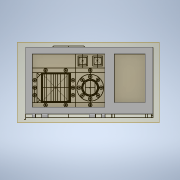
# Autodesk Inventor part: authentication panel v1.1
Saved by Autodesk Inventor 2022 (Build 260153000, 153)
## iProperties
Created: 2022-05-25
Part Number: authentication panel v1.1
Material: Generic
Document SubType Name: Modeling
Designer: alecw
Density: 1 g/cm^3
Appearance: Default
Author: alecw
Autodesk Inventor part; units mm, degrees
ref_plane "YZ Plane" through (0, 0, 0) normal (1, 0, 0) x (0, 1, 0)
ref_plane "XZ Plane" through (0, 0, 0) normal (0, 1, 0) x (-1, 0, 0)
ref_plane "Backplate Depth" through (0, 0, -3.2) normal (0, 0, 1) x (1, 0, 0)
sketch "Sketch2" plane through (0, 0, 0) normal (0, 0, 1) x (1, 0, 0)
  line L0 (0, 0) -> (45, 0)
  line L1 (45, 0) -> (45, 65)
  line L2 (45, 65) -> (0, 65)
  line L3 (0, 65) -> (0, 0)
  line L4 (0, 0) -> (-8.8, 0)
  line L5 (-8.8, 0) -> (-12, 0)
  line L6 (-12, 0) -> (-42, 0)
  line L7 (-42, 0) -> (-54.8, 0)
  line L8 (-54.8, 0) -> (-99.5, 0)
  line L9 (-99.5, 0) -> (-105.9, 0)
  line L10 (-105.9, 0) -> (-114.7, 0)
  line L11 (-114.7, 0) -> (-114.7, 40.1)
  line L12 (-114.7, 40.1) -> (0, 40.1)
  line L13 (-114.7, 0) -> (0, 0)
  line L14 (-105.9, 0) -> (-105.9, 40.1)
  line L15 (-8.8, 40.1) -> (-8.8, 0)
  line L16 (-48.4, 0) -> (-8.8, 0)
  line L17 (0, 65) -> (-114.7, 65)
  line L18 (-114.7, 65) -> (-114.7, 40.1)
  line L19 (45, 0) -> (48.2, 0)
  line L20 (0, 65) -> (0, 68.2)
  line L21 (0, 68.2) -> (48.2, 68.2)
  line L22 (48.2, 68.2) -> (48.2, 0)
  line L23 (-54.8, 0) -> (-48.4, 0)
  line L24 (-42, 0) -> (-48.4, 0)
  line L25 (-48.4, 0) -> (-48.4, 40.1)
  line L26 (-105.9, 40.1) -> (-105.9, 33.7)
  line L27 (-105.9, 40.1) -> (-93.1, 40.1)
  line L28 (-105.9, 0) -> (-48.4, 0)
  line L29 (-99.5, 0) -> (-88.19, 0)
  line L30 (-88.19, 0) -> (-79.22, 0)
  line L31 (-54.8, 0) -> (-54.8, 40.1)
  line L32 (-99.5, 0) -> (-99.5, 40.1)
  line L33 (-54.8, 40.1) -> (-56.9213, 37.9787)
  line L34 (-54.8, 40.1) -> (-51.8, 40.1) construction
  line L35 (-56.9213, 37.9787) -> (-54.8, 35.8574)
  line L36 (-56.9213, 37.9787) -> (-59.0426, 40.1)
  line L37 (-54.8, 0) -> (-57.6284, 2.8284)
  line L38 (-54.8, 0) -> (-50.8, 0) construction
  line L39 (-99.5, 40.1) -> (-95.9645, 36.5645)
  line L40 (-99.5, 40.1) -> (-94.5, 40.1) construction
  line L41 (-95.9645, 36.5645) -> (-92.4289, 40.1)
  line L42 (-95.9645, 36.5645) -> (-99.5, 33.0289)
  line L43 (-99.5, 0) -> (-95.9645, 3.5355)
  line L44 (-99.5, 0) -> (-94.5, 0) construction
  line L45 (-95.9645, 3.5355) -> (-92.4289, 0)
  line L46 (-95.9645, 3.5355) -> (-99.5, 7.0711)
  line L47 (-48.4, 0) -> (-48.4, -6.4)
  line L48 (-48.4, -6.4) -> (-105.9, -6.4)
  line L49 (-105.9, -6.4) -> (-105.9, 0)
  line L50 (-105.9, 40.1) -> (-105.9, 46.5)
  line L51 (-48.4, 40.1) -> (-48.4, 46.5)
  line L52 (-48.4, 46.5) -> (-105.9, 46.5)
  line L53 (-88.19, 0) -> (-86.59, 0)
  line L54 (-88.19, 0) -> (-89.79, 0)
  line L55 (-89.79, 0) -> (-86.59, 0)
  line L56 (-86.59, 0) -> (-86.59, 40.1)
  line L57 (-86.59, 40.1) -> (-89.79, 40.1)
  line L58 (-89.79, 40.1) -> (-89.79, 0)
  line L59 (-80.82, 40.1) -> (-80.82, 0)
  line L60 (-77.62, 0) -> (-77.62, 40.1)
  line L61 (-71.85, 40.1) -> (-71.85, 0)
  line L62 (-68.65, 0) -> (-68.65, 40.1)
  line L63 (-62.88, 40.1) -> (-62.88, 0)
  line L64 (-59.68, 0) -> (-59.68, 40.1)
  line L65 (0, 0) -> (0, -6.4)
  line L66 (0, -6.4) -> (0, -15.2)
  line L67 (-114.7, 0) -> (-114.7, -6.4)
  line L68 (-114.7, -6.4) -> (-114.7, -15.2)
  line L69 (-114.7, -15.2) -> (0, -15.2)
  line L70 (0, -15.2) -> (48.2, -15.2)
  line L71 (48.2, -15.2) -> (48.2, 0)
  line L72 (-28.6, 40.1) -> (-28.6, 0)
  circle A0 centre (-28.6, 20.05) radius 9.5
  circle A1 centre (-28.6, 20.05) radius 10.5
  line L73 (-28.6, 29.55) -> (-27.4024, 29.4742)
  line L74 (-27.4024, 29.4742) -> (-27.3391, 30.474)
  line L75 (-28.6, 29.55) -> (-29.7976, 29.4742)
  line L76 (-29.7976, 29.4742) -> (-29.8609, 30.474)
  line L77 (-105.9, 46.5) -> (-114.7, 46.5)
  line L78 (-105.9, -6.4) -> (-114.7, -6.4)
  line L79 (-48.4, -6.4) -> (0, -6.4)
  line L80 (-28.6, 20.05) -> (-35, 20.05)
  line L81 (-28.6, 20.05) -> (-22.2, 20.05)
  circle A2 centre (-28.6, 20.05) radius 17.9
  line L82 (-77.62, 40.1) -> (-71.85, 40.1)
  line L83 (-88.19, 40.1) -> (-92.19, 40.1)
  line L84 (-92.19, 40.1) -> (-93.79, 40.1)
  line L85 (-74.735, 0) -> (-74.735, 40.1)
  line L86 (-92.135, 38.25) -> (-57.335, 38.25)
  line L87 (-57.335, 38.25) -> (-57.335, 1.85)
  line L88 (-57.335, 1.85) -> (-92.135, 1.85)
  line L89 (-92.135, 1.85) -> (-92.135, 38.25)
  line L90 (-92.135, 38.25) -> (-57.335, 1.85) construction
  line L91 (-57.335, 38.25) -> (-92.135, 1.85) construction
  line L92 (-74.735, 38.25) -> (-74.735, 40.1)
  line L93 (-18.1, 20.05) -> (-17.1, 20.05)
  circle A3 centre (-28.6, 20.05) radius 11.5
  line L94 (-17.1, 20.05) -> (-10.7, 20.05)
  circle A4 centre (-13.9, 20.05) radius 0.9
  line L95 (-54.8, 40.1) -> (-48.4, 40.1)
  line L96 (-89.79, 38.25) -> (-86.59, 38.25)
  line L97 (-59.68, 38.25) -> (-62.88, 38.25)
  line L98 (-92.135, 20.05) -> (-57.335, 20.05)
  circle A5 centre (-18.2055, 30.4445) radius 0.9
  circle A6 centre (-28.6, 34.75) radius 0.9
  circle A7 centre (-38.9945, 30.4445) radius 0.9
  circle A8 centre (-43.3, 20.05) radius 0.9
  circle A9 centre (-38.9945, 9.6555) radius 0.9
  circle A10 centre (-28.6, 5.35) radius 0.9
  circle A11 centre (-18.2055, 9.6555) radius 0.9
  line L99 (-57.6284, 2.8284) -> (-54.8, 5.6569)
  line L100 (-57.6284, 2.8284) -> (-60.4569, 0)
  line L101 (-99.5, 20.05) -> (-105.9, 20.05)
  circle A12 centre (-102.7, 20.05) radius 0.9
  line L102 (-54.8, 20.05) -> (-48.4, 20.05)
  circle A13 centre (-51.6, 20.05) radius 0.9
  line L103 (0, -15.2) -> (0, -20)
  line L104 (0, -20) -> (-114.7, -20)
  line L105 (-114.7, -20) -> (-114.7, -15.2)
  line L106 (-88.19, 40.1) -> (-88.19, 43.3)
  circle A14 centre (-88.19, 43.3) radius 0.9
  circle A15 centre (-61.28, 43.3) radius 0.9
  circle A16 centre (-88.19, -3.2) radius 0.9
  circle A17 centre (-61.28, -3.2) radius 0.9
  line L107 (-102.7, 20.05) -> (-102.7, 0)
  circle A18 centre (-102.7, 10.025) radius 0.9
  circle A19 centre (-102.7, 30.075) radius 0.9
  circle A20 centre (-51.6, 30.075) radius 0.9
  circle A21 centre (-51.6, 10.025) radius 0.9
  line L108 (0, -20) -> (48.2, -20)
  line L109 (48.2, -20) -> (48.2, -15.2)
  line L110 (0, 65) -> (0, 73.8)
  line L111 (0, 73.8) -> (-114.7, 73.8)
  line L112 (-114.7, 73.8) -> (-114.7, 65)
  line L113 (-105.9, -20) -> (-105.9, 73.8)
  line L114 (-8.8, -20) -> (-8.8, 73.8)
  line L115 (-28.6, 40.1) -> (-48.4, 40.1)
  line L116 (-28.6, 40.1) -> (-8.8, 40.1)
  line L117 (-48.4, 46.5) -> (-28.6, 46.5)
  line L118 (-28.6, 46.5) -> (-8.8, 46.5)
  line L119 (-38.5, 46.5) -> (-38.5, 65)
  line L120 (-18.7, 46.5) -> (-18.7, 65)
  line L121 (-13.7, 60.75) -> (-23.7, 60.75)
  line L122 (-23.7, 60.75) -> (-23.7, 50.75)
  line L123 (-23.7, 50.75) -> (-13.7, 50.75)
  line L124 (-13.7, 50.75) -> (-13.7, 60.75)
  line L125 (-13.7, 60.75) -> (-23.7, 50.75) construction
  line L126 (-23.7, 60.75) -> (-13.7, 50.75) construction
  line L127 (-33.5, 50.75) -> (-43.5, 50.75)
  line L128 (-43.5, 50.75) -> (-43.5, 60.75)
  line L129 (-43.5, 60.75) -> (-33.5, 60.75)
  line L130 (-33.5, 60.75) -> (-33.5, 50.75)
  line L131 (-33.5, 50.75) -> (-43.5, 60.75) construction
  line L132 (-43.5, 50.75) -> (-33.5, 60.75) construction
  line L133 (-32, 49.25) -> (-45, 49.25)
  line L134 (-45, 49.25) -> (-45, 62.25)
  line L135 (-45, 62.25) -> (-32, 62.25)
  line L136 (-32, 62.25) -> (-32, 49.25)
  line L137 (-32, 49.25) -> (-45, 62.25) construction
  line L138 (-45, 49.25) -> (-32, 62.25) construction
  line L139 (-12.2, 62.25) -> (-25.2, 62.25)
  line L140 (-25.2, 62.25) -> (-25.2, 49.25)
  line L141 (-25.2, 49.25) -> (-12.2, 49.25)
  line L142 (-12.2, 49.25) -> (-12.2, 62.25)
  line L143 (-12.2, 62.25) -> (-25.2, 49.25) construction
  line L144 (-25.2, 62.25) -> (-12.2, 49.25) construction
  line L145 (-33.5, 50.75) -> (-33.5, 49.25)
  line L146 (-43.5, 50.75) -> (-43.5, 49.25)
  circle A22 centre (-88.19, 43.3) radius 2.4
  circle A23 centre (-61.28, 43.3) radius 2.4
  circle A24 centre (-51.6, 30.075) radius 2.4
  circle A25 centre (-51.6, 20.05) radius 2.4
  circle A26 centre (-51.6, 10.025) radius 2.4
  circle A27 centre (-61.28, -3.2) radius 2.4
  circle A28 centre (-88.19, -3.2) radius 2.4
  circle A29 centre (-102.7, 10.025) radius 2.4
  circle A30 centre (-102.7, 20.05) radius 2.4
  circle A31 centre (-102.7, 30.075) radius 2.4
  circle A32 centre (-13.9, 20.05) radius 2.4
  circle A33 centre (-18.2055, 30.4445) radius 2.4
  circle A34 centre (-28.6, 34.75) radius 2.4
  circle A35 centre (-38.9945, 30.4445) radius 2.4
  circle A36 centre (-43.3, 20.05) radius 2.4
  circle A37 centre (-38.9945, 9.6555) radius 2.4
  circle A38 centre (-28.6, 5.35) radius 2.4
  circle A39 centre (-18.2055, 9.6555) radius 2.4
  line L147 (-114.7, -20) -> (-114.7, -22.4)
  line L148 (-114.7, -22.4) -> (-117.1, -22.4)
  line L149 (-114.7, -15.2) -> (-114.7, -12.8)
  line L150 (-114.7, -12.8) -> (-112.3, -12.8)
  line L151 (0, 73.8) -> (-2.4, 73.8)
  line L152 (-2.4, 73.8) -> (-2.4, 71.4)
  line L153 (-112.3, -12.8) -> (-112.3, 71.4)
  line L154 (-112.3, 71.4) -> (-2.4, 71.4)
  line L155 (-2.4, 71.4) -> (-2.4, -12.8)
  line L156 (-2.4, -12.8) -> (-112.3, -12.8)
  line L157 (-2.4, -15.2) -> (-2.4, -12.8)
  line L158 (-28.6, -6.4) -> (-28.6, 0)
  circle A40 centre (-28.6, -3.2) radius 2.4
  circle A41 centre (-28.6, -3.2) radius 0.9
  line L159 (-28.6, 40.1) -> (-28.6, 46.5)
  circle A42 centre (-28.6, 43.3) radius 0.9
  circle A43 centre (-28.6, 43.3) radius 2.4
  line L160 (-105.9, 65) -> (-105.9, 71.4)
  circle A44 centre (-109.1, 68.2) radius 0.9
  circle A45 centre (-109.1, 68.2) radius 2
  line L161 (-8.8, 65) -> (-2.4, 65)
  line L162 (-8.8, -6.4) -> (-8.8, -12.8)
  line L163 (-105.9, 65) -> (-112.3, 65)
  line L164 (-105.9, 65) -> (-105.9, 71.4)
  line L165 (-105.9, 68.2) -> (-109.1, 68.2)
  line L166 (-109.1, 65) -> (-109.1, 68.2)
  line L167 (-105.9, -6.4) -> (-105.9, -12.8)
  circle A46 centre (-57.35, 68.2) radius 2
  circle A47 centre (-57.35, 68.2) radius 0.9
  circle A48 centre (-5.6, 68.2) radius 2
  circle A49 centre (-5.6, 68.2) radius 0.9
  circle A50 centre (-109.1, -9.6) radius 2
  circle A51 centre (-109.1, -9.6) radius 0.9
  circle A52 centre (-57.35, -9.6) radius 2
  circle A53 centre (-57.35, -9.6) radius 0.9
  circle A54 centre (-5.6, -9.6) radius 2
  circle A55 centre (-5.6, -9.6) radius 0.9
  line L168 (-105.9, -6.4) -> (-105.9, 65)
  line L169 (-105.9, 29.3) -> (-112.3, 29.3)
  circle A56 centre (-109.1, 29.3) radius 2
  circle A57 centre (-109.1, 29.3) radius 0.9
  circle A58 centre (-5.6, 29.3) radius 0.9
  circle A59 centre (-5.6, 29.3) radius 2
  line L170 (-105.9, 29.3) -> (-105.9, 65)
  line L171 (-8.8, 65) -> (-105.9, 65)
  line L172 (-57.35, 65) -> (-109.1, 65)
  circle A60 centre (-109.1, 68.2) radius 1.6
  circle A61 centre (-97.6, 68.2) radius 1.6
  circle A62 centre (-86.1, 68.2) radius 1.6
  circle A63 centre (-74.6, 68.2) radius 1.6
  circle A64 centre (-63.1, 68.2) radius 1.6
  circle A65 centre (-51.6, 68.2) radius 1.6
  circle A66 centre (-40.1, 68.2) radius 1.6
  circle A67 centre (-28.6, 68.2) radius 1.6
  circle A68 centre (-17.1, 68.2) radius 1.6
  circle A69 centre (-109.1, 57.0857) radius 1.6
  circle A70 centre (-109.1, 45.9714) radius 1.6
  circle A71 centre (-109.1, 34.8571) radius 1.6
  circle A72 centre (-109.1, 23.7429) radius 1.6
  circle A73 centre (-109.1, 12.6286) radius 1.6
  circle A74 centre (-109.1, 1.5143) radius 1.6
  line L173 (-57.35, 65) -> (-57.35, 71.4)
  circle A75 centre (-97.6, -9.6) radius 1.6
  circle A76 centre (-86.1, -9.6) radius 1.6
  circle A77 centre (-74.6, -9.6) radius 1.6
  circle A78 centre (-63.1, -9.6) radius 1.6
  circle A79 centre (-51.6, -9.6) radius 1.6
  circle A80 centre (-40.1, -9.6) radius 1.6
  circle A81 centre (-28.6, -9.6) radius 1.6
  circle A82 centre (-17.1, -9.6) radius 1.6
  circle A83 centre (-5.6, 57.0857) radius 1.6
  circle A84 centre (-5.6, 45.9714) radius 1.6
  circle A85 centre (-5.6, 34.8571) radius 1.6
  circle A86 centre (-5.6, 23.7429) radius 1.6
  circle A87 centre (-5.6, 12.6286) radius 1.6
  circle A88 centre (-5.6, 1.5143) radius 1.6
  line L174 (-48.4, 46.5) -> (-48.4, 65)
  line L175 (-92.135, 38.25) -> (-92.985, 38.25)
  line L176 (-92.985, 38.25) -> (-92.985, 39.1)
  line L177 (-56.485, 1) -> (-92.985, 1)
  line L178 (-92.985, 1) -> (-92.985, 39.1)
  line L179 (-92.985, 39.1) -> (-56.485, 39.1)
  line L180 (-56.485, 39.1) -> (-56.485, 1)
  line L181 (-56.485, 1) -> (-92.985, 39.1) construction
  line L182 (-92.985, 1) -> (-56.485, 39.1) construction
  line L183 (-92.985, 39.1) -> (-92.985, 40.1)
  line L184 (-92.985, 40.1) -> (-93.985, 40.1)
  line L185 (-55.485, 0) -> (-93.985, 0)
  line L186 (-93.985, 0) -> (-93.985, 40.1)
  line L187 (-93.985, 40.1) -> (-55.485, 40.1)
  line L188 (-55.485, 40.1) -> (-55.485, 0)
  line L189 (-55.485, 0) -> (-93.985, 40.1) construction
  line L190 (-93.985, 0) -> (-55.485, 40.1) construction
  line L191 (48.2, -20) -> (53.2, -20)
  line L192 (53.2, -20) -> (53.2, 68.2)
  line L193 (53.2, 68.2) -> (48.2, 68.2)
  line L194 (53.2, -20) -> (55.2, -20)
  line L195 (55.2, -20) -> (55.2, 68.2)
  line L196 (55.2, 68.2) -> (53.2, 68.2)
  line L197 (53.2, 65) -> (55.2, 65)
  line L198 (53.2, -20) -> (53.2, -16.8)
  line L199 (53.2, -16.8) -> (55.2, -16.8)
  line L200 (-8.8, -20) -> (-105.9, -20)
  line L201 (-105.9, -20) -> (-101.9, -20)
  line L202 (-57.35, -20) -> (-57.35, -15.2)
  line L203 (-101.9, -20) -> (-101.4, -20)
  line L204 (-101.4, -20) -> (-93.4, -20)
  line L205 (-93.4, -20) -> (-93.4, -15.2)
  line L206 (-101.9, -20) -> (-101.9, -15.2)
  line L207 (-101.4, -20) -> (-101.4, -15.2)
  line L208 (-93.4, -20) -> (-92.9, -20)
  line L209 (-92.9, -20) -> (-84.9, -20)
  line L210 (-84.9, -20) -> (-84.9, -15.2)
  line L211 (-8.8, -20) -> (-12.8, -20)
  line L212 (-12.8, -20) -> (-13.3, -20)
  line L213 (-13.3, -20) -> (-21.3, -20)
  line L214 (-21.3, -20) -> (-21.3, -15.2)
  line L215 (-12.8, -20) -> (-12.8, -15.2)
  line L216 (-13.3, -20) -> (-13.3, -15.2)
  line L217 (-21.3, -20) -> (-21.8, -20)
  line L218 (-21.8, -20) -> (-29.8, -20)
  line L219 (-29.8, -20) -> (-29.8, -15.2)
  line L220 (-57.35, 73.8) -> (-57.35, 75.8)
  line L221 (-57.35, 75.8) -> (-77.35, 75.8)
  line L222 (-77.35, 75.8) -> (-79.35, 73.8)
  line L223 (-77.35, 75.8) -> (-74.5216, 75.8) construction
  line L224 (-57.35, 75.8) -> (-37.35, 75.8)
  line L225 (-37.35, 75.8) -> (-35.35, 73.8)
  line L226 (0, 73.8) -> (55.2, 73.8)
  line L227 (55.2, 73.8) -> (55.2, 68.2)
  line L228 (0, 73.8) -> (0.5, 73.8)
  line L229 (0.5, 73.8) -> (0.5, -20)
  line L230 (53.2, 68.2) -> (53.2, 73.8)
  line L231 (48.2, -15.2) -> (55.2, -15.2)
  line L232 (-92.9, -20) -> (-92.9, -15.2)
  line L233 (-21.8, -20) -> (-21.8, -15.2)
  line L234 (0.5, -15.2) -> (0.5, -12)
  line L235 (0.5, -12) -> (48.2, -12)
  line L236 (0.5, -15.2) -> (0.5, -12)
  line L237 (0.5, -12) -> (48.2, -12)
  line L238 (45, 0) -> (45, -15.2)
  line L239 (45, 68.2) -> (45, 65)
  line L240 (48.2, 65) -> (45, 65)
  line L241 (0.5, -15.2) -> (3.7, -15.2)
  line L242 (3.7, -15.2) -> (3.7, 65)
  line L243 (48.2, 68.2) -> (48.2, 73.8)
  line L244 (45, 68.2) -> (45, 73.8)
  line L245 (45, -15.2) -> (45, -20)
  line L246 (3.7, -15.2) -> (3.7, -20)
  line L247 (3.7, 65) -> (3.7, 73.8)
  line L248 (48.2, -12) -> (55.2, -12)
  line L249 (55.2, 65) -> (48.2, 65)
  line L250 (-35, 20.05) -> (-35, 13.0293)
  line L251 (-35, 20.05) -> (-35, 27.0707)
  line L252 (-22.2, 20.05) -> (-22.2, 27.0707)
  line L253 (-22.2, 20.05) -> (-22.2, 13.0293)
  line L254 (0, -6.4) -> (55.2, -6.4)
  line L255 (0, 0) -> (55.2, 0)
  point P0 (-74.735, 20.05)
  point P1 (-74.735, 20.05)
  point P2 (-18.7, 55.75)
  point P3 (-38.5, 55.75)
  point P4 (-112.3, 0)
  point P5 (-8.8, 71.4)
  point P6 (0.5, 0)
  point P7 (53.2, -15.2)
  point P8 (-8.8, -15.2)
  point P9 (-105.9, -15.2)
  point P10 (3.7, 0)
  point P11 (53.2, 0)
  dimension "d1" = 45
  dimension "d2" = 65
  dimension "d3" = 8.8
  dimension "d4" = 3.2
  dimension "d5" = 30
  dimension "d6" = 12.8
  dimension "d7" = 44.7
  dimension "d11" = 40.1
  dimension "d15" = 3.2
  dimension "d16" = 3.2
  dimension "d21" = 11.31
  dimension "d22" = 8.97
  dimension "d23" = 3
  dimension "d24" = 135
  dimension "d25" = 4
  dimension "d26" = 135
  dimension "d27" = 5
  dimension "d28" = 45
  dimension "d29" = 5
  dimension "d30" = 45
  dimension "d33" = 6.4
  dimension "d34" = 1.6
  dimension "d35" = 1.6
  dimension "d38" = 8.97
  dimension "d43" = 3.2
  dimension "d45" = 19
  dimension "d46" = 21
  dimension "d47" = 1.2
  dimension "d48" = 6.4
  dimension "d49" = 6.4
  dimension "d53" = 4
  dimension "d54" = 1.6
  dimension "d55" = 34.8
  dimension "d56" = 36.4
  dimension "d59" = 1
  dimension "d61" = 6.4
  dimension "d62" = 1.8
  dimension "d68" = 360
  dimension "d70" = 1.8
  dimension "d71" = 1.8
  dimension "d72" = 4.8
  dimension "d74" = 3.2
  dimension "d75" = 1.8
  dimension "d76" = 1.8
  dimension "d79" = 51.1
  dimension "d86" = 10
  dimension "d88" = 13
  dimension "d89" = 4.8
  dimension "d92" = 360
  dimension "d98" = 2.4
  dimension "d99" = 2.4
  dimension "d100" = 2.4
  dimension "d101" = 2.4
  dimension "d102" = 2.4
  dimension "d103" = 2.4
  dimension "d104" = 2.4
  dimension "d105" = 1.8
  dimension "d106" = 4
  dimension "d109" = 51.75
  dimension "d116" = 77.8
  dimension "d123" = 38.9
  dimension "d128" = 3.2
  dimension "d131" = 11.5
  dimension "d138" = 11.1143
  constraints: 508 end point, 107 point on line, 88 centre point, 54 perpendicular, 48 horizontal, 46 midpoint, 37 vertical, 35 parallel, 32 symmetric about line, 27 coincident, 16 collinear, 16 equal radius, 15 horizontal alignment, 10 point on circle, 5 equal length, 134 other
  measures "d1" distance of L2.end L1.end
  measures "d2" distance of L1.end L0.end
  measures "d3" distance of L0.start L4.end
  measures "d4" distance of L4.end L5.end
  measures "d5" distance of L5.end L6.end
  measures "d6" distance of L6.end L7.end
  measures "d7" distance of L7.end L8.end
  measures "d11" distance of L10.end L11.end
  measures "d15" distance of L0.end L19.end
  measures "d16" distance of L2.end L20.end
  measures "d21" distance of L8.end L29.end
  measures "d22" distance of L29.end L30.end
  measures "d23" distance of L31.end L33.end
  measures "d24" angle of L33 L34
  measures "d25" distance of L7.end L37.end
  measures "d26" angle of L38 L37
  measures "d27" distance of L32.end L39.end
  measures "d28" angle of L39 L40
  measures "d29" distance of L8.end L43.end
  measures "d30" angle of L44 L43
  measures "d33" distance of L25.end L51.end
  measures "d34" distance of L29.end L53.end
  measures "d35" distance of L29.end L54.end
  measures "d38" distance of L57.end L59.start
  measures "d43" distance between parallel lines of L56 L58
  measures "d45" diameter of A0
  measures "d46" diameter of A1
  measures "d47" distance of L73.start L73.end
  measures "d48" distance of L80.start L80.end
  measures "d49" distance of L80.start L81.end
  measures "d53" distance of L83.start L83.end
  measures "d54" distance of L83.end L84.end
  measures "d55" distance of L87.end L88.end
  measures "d56" distance of L86.end L87.end
  measures "d59" distance of L93.start L93.end
  measures "d61" distance of L94.start L94.end
  measures "d62" diameter of A4
  measures "d70" diameter of A12
  measures "d71" diameter of A13
  measures "d72" distance of L66.end L103.end
  measures "d74" distance of L83.start L106.end
  measures "d75" diameter of A14
  measures "d76" diameter of A18
  measures "d79" distance of A19.centre A20.centre
  measures "d86" distance of L128.end L129.end
  measures "d88" distance of L133.end L134.end
  measures "d89" diameter of A22
  measures "d98" distance of L104.end L147.end
  measures "d99" distance of L147.end L148.end
  measures "d100" distance of L68.end L149.end
  measures "d101" distance of L149.end L150.end
  measures "d102" distance of L110.end L151.end
  measures "d103" distance of L151.end L152.end
  measures "d104" distance of L157.start L155.end
  measures "d105" diameter of A44
  measures "d106" diameter of A45
  measures "d109" distance of L165.end A46.centre
  measures "d116" distance of L165.end A50.centre
  measures "d123" distance of L165.end A56.centre
  measures "d128" diameter of A60
  measures "d131" distance of A60.centre A61.centre
  measures "d138" distance of A60.centre A69.centre
ref_plane "Face Plate Start" through (0, 0, 5) normal (0, 0, 1) x (1, 0, 0)
ref_plane "TPU Seal Start" through (0, 0, 4) normal (0, 0, 1) x (1, 0, 0)
ref_plane "Face Plate End" through (0, 0, 8.2) normal (0, 0, 1) x (1, 0, 0)
ref_plane "Cover Clearance" through (0, 0, 11.2) normal (0, 0, 1) x (1, 0, 0)
ref_plane "Cover End" through (0, 0, 13.6) normal (0, 0, 1) x (1, 0, 0)
extrude "backplate" add sketch "Sketch2" against normal up to surface (3.2 mm away) contours L3 L2 L229 L0 | L4 L155 L12 L3 | L65 L79 L155 L4 | L0 L229 L254 L65 | L229 L2 L242 L0 | L0 L242 L254 L229 | L12 L155 L17 L3 | L155 L79 L114 L4 A88 | L4 A88 L15 L12 L155 | L254 L229 L70 L66 | L66 L69 L157 L155 L79 | L242 L2 L1 L0 | L0 L238 L254 L242 | L229 L21 L247 L2 | L2 L20 L21 L229 | L254 L242 L235 L229 | L17 L155 L152 L111 L110 L20 | L12 L114 L17 L155 | A88 L4 | L4 A88 | L155 L156 L114 L79 | L1 L240 L22 L19 | L19 L71 L254 L238 | L254 L238 L235 L242 | L247 L21 L239 L2 | L229 L226 L247 L21 | L21 L110 L226 L229 | L235 L242 L70 L229 | L17 L114 L154 L155 | L15 L5 L6 L72 A2 L12 | L12 L159 A43 L118 L114 | L114 L156 L113 L48 L79 | L79 L158 A40 L6 L5 L114 | L157 L69 L114 L156 | L239 L21 L22 L240 | L255 L192 L254 L71 | L22 L249 L192 L255 | L254 L71 L235 L238 | L235 L238 L70 L242 | L247 L226 L244 L21 | L114 L118 L120 L141 L142 L139 L17 | L17 L173 A46 L154 L114 | L154 L114 L111 L152 | L72 A2 L6 L7 L25 L12 | L12 L51 L117 L159 A43 | L79 L47 L7 L6 L158 A40 | L114 L69 L113 L156 | L244 L226 L243 L21 | L22 L193 L192 L249 | L254 L192 L248 L71 | L235 L71 L70 L238 | L120 L139 L140 L141 L118 L117 L119 L133 L136 L135 L17 | L154 L113 L111 L114 | L25 L102 A25 L31 L12 | L12 L50 L52 L51 | A2 L94 A32 A3 L72 A34 | L72 A34 A3 A38 A2 | A43 L159 A42 | L159 A42 A43 | L48 L49 L9 L8 L7 L47 | A40 L158 A41 | L158 A41 A40 | L156 L153 L78 L113 | L113 L69 L68 L150 L156 | L243 L226 L230 L193 | L248 L192 L231 L71 | L119 L135 L134 L133 L117 L174 L17 | L139 L142 L141 L120 L123 L124 L121 | L120 L121 L122 L123 L141 L140 L139 | L173 A46 L17 L113 L154 | L33 L188 L12 | L31 L35 L188 L33 | L25 L7 L31 L102 A25 | L52 L113 L17 L174 | A34 L72 A6 | L72 A6 A34 | A2 L72 A38 A3 L94 A32 | A42 L159 | L159 A42 | L78 L153 L10 A74 L49 | A41 L158 | L158 A41 | L150 L68 L78 L153 | L135 L136 L133 L145 L130 L129 L119 | L119 L129 L128 L146 L133 L134 L135 | L121 L124 L123 L120 | L120 L123 L122 L121 | L154 L153 L17 L112 L111 L113 | L113 L165 A45 L166 L17 L153 L154 | L173 A47 A46 | A46 L173 A47 | L188 L33 L180 L179 L36 L12 | L31 L99 L188 L35 | L188 L35 L180 L33 | A25 L102 A13 | L102 A13 A25 | L50 L12 L153 L77 A70 | L77 A70 L153 L17 L113 | A6 L72 | L72 A6 | A32 L94 A4 | L94 A4 A32 | A38 L72 A10 | L72 A10 A38 | L37 L188 L99 L31 | L8 L188 L37 | L14 L101 A30 L107 A29 L9 | L10 A74 L153 L169 A56 L14 | L78 L67 L10 L153 | L129 L130 L127 L119 | L119 L127 L128 L129 | L113 L17 L166 A45 L165 | L173 A47 | A47 L173 | L36 L179 L64 L12 | L188 L99 L180 L35 | L180 L35 L33 | L33 L36 L179 L180 | A13 L102 | L102 A13 | L14 L169 A56 L153 L12 | L12 L32 L101 A30 L14 | A70 L77 | L77 A70 | L133 L146 L127 L119 | L119 L127 L145 L133 | A3 L93 A1 L72 | L72 A1 A3 | A4 L94 | L94 A4 | A10 L72 | L72 A10 | L8 L64 L100 L177 L180 L37 L188 | L37 L180 L99 L188 | L107 A29 A30 L101 L32 L9 | A74 L10 | L10 A74 | L10 L11 L12 L153 | L165 A60 L166 A45 | A45 L166 A60 L165 | L153 L77 L18 L17 | L64 L179 L63 L12 | L36 L35 L180 L99 L87 L86 L64 L179 | L39 L42 L32 | L12 L186 L41 L39 | L12 L18 L77 L153 | A1 L74 A0 L72 | L72 A0 L76 A1 | A3 L72 A1 L93 | L8 L100 L64 | L180 L177 L100 L88 L87 L37 | L37 L87 L99 L180 | L43 L45 L186 L8 | L32 L46 L43 | A29 L107 A18 | L107 A18 A29 | A30 L101 A12 | L101 A12 L107 A30 | A60 L166 A44 L165 | L165 A44 L166 A60 | L63 L179 L62 L12 | L64 L86 L63 L179 | L12 L183 L41 L186 | L42 L41 L186 L45 L46 L32 | L73 A0 L252 L81 L72 | L75 A0 | A0 L73 | L72 L80 L251 A0 L75 | A1 L72 A0 L74 | L76 A0 L72 A1 | L8 L63 L177 L64 L100 | L64 L177 L100 | L87 L88 L100 L37 | L37 L99 L87 | L186 L45 L8 | A18 L107 | L107 A18 | A56 L169 A57 | L169 A57 A56 | A12 L101 | L101 L107 A12 | A30 L107 A12 L101 | L165 L166 A44 | A44 L166 L165 | L62 L179 L61 L12 | L63 L86 L62 L179 | L86 L87 L98 L64 | L64 L98 L63 L86 | L99 L100 L88 L64 L98 L87 | L41 L183 L176 L178 L177 L58 L8 L45 L186 | L81 L253 A0 L72 | L72 A0 L250 L80 | L8 L62 L177 L63 | L177 L63 L88 L64 | L64 L88 L100 L177 | A57 L169 | L169 A57 | L101 A12 L107 | L61 L179 L85 L12 | L62 L86 L61 L179 | L63 L98 L62 L86 | L64 L88 L63 L98 | L183 L12 L41 | L41 L12 L58 L179 L183 | L250 A0 L251 | L252 A0 L253 | L8 L61 L177 L62 | L177 L62 L88 L63 | L58 L177 L56 L8 | L85 L179 L60 L12 | L61 L86 L85 L179 | L62 L98 L61 L86 | L63 L88 L62 L98 | L179 L58 L86 L175 L176 | L8 L85 L177 L61 | L177 L61 L88 L62 | L177 L178 L175 L89 L88 L58 | L58 L88 L56 L177 | L60 L179 L59 L12 | L85 L86 L60 L179 | L61 L98 L85 L86 | L62 L88 L61 L98 | L179 L56 L86 L58 | L58 L12 L56 L179 | L8 L60 L177 L85 | L177 L85 L88 L61 | L56 L177 L59 L8 | L88 L89 L98 L58 | L58 L98 L56 L88 | L56 L88 L59 L177 | L59 L179 L56 L12 | L60 L86 L59 L179 | L85 L98 L60 L86 | L61 L88 L85 L98 | L86 L58 L98 L89 | L86 L56 L98 L58 | L179 L59 L86 L56 | L8 L59 L177 L60 | L177 L60 L88 L85 | L56 L98 L59 L88 | L59 L88 L60 L177 | L60 L98 L59 L86 | L85 L88 L60 L98 | L86 L59 L98 L56 | L59 L98 L60 L88 | A5 | A7 | A8 | A9 | A11 | A14 | A15 | A16 | A17 | A19 | A20 | A21 | A22 | A23 | A24 | A26 | A27 | A28 | A31 | A33 | A35 | A36 | A37 | A39 | A48 | A49 | A50 | A51 | A52 | A53 | A54 | A55 | A58 | A59 | A61 | A62 | A63 | A64 | A65 | A66 | A67 | A68 | A69 | A71 | A72 | A73 | A75 | A76 | A77 | A78 | A79 | A80 | A81 | A82 | A83 | A84 | A85 | A86 | A87
extrude "enclosure walls" add sketch "Sketch2" along normal up to surface (5 mm away) contours L3 L2 L229 L0 | L4 L155 L12 L3 | L65 L79 L155 L4 | L0 L229 L254 L65 | L229 L2 L242 L0 | L0 L242 L254 L229 | L12 L155 L17 L3 | L155 L79 L114 L4 A88 | L4 A88 L15 L12 L155 | L254 L229 L70 L66 | L66 L69 L157 L155 L79 | L0 L238 L254 L242 | L229 L21 L247 L2 | L2 L20 L21 L229 | L254 L242 L235 L229 | L17 L155 L152 L111 L110 L20 | L12 L114 L17 L155 | A88 L4 | L4 A88 | L155 L156 L114 L79 | L1 L240 L22 L19 | L19 L71 L254 L238 | L254 L238 L235 L242 | L247 L21 L239 L2 | L229 L226 L247 L21 | L21 L110 L226 L229 | L235 L242 L70 L229 | L17 L114 L154 L155 | L114 L156 L113 L48 L79 | L157 L69 L114 L156 | L239 L21 L22 L240 | L255 L192 L254 L71 | L22 L249 L192 L255 | L254 L71 L235 L238 | L235 L238 L70 L242 | L247 L226 L244 L21 | L17 L173 A46 L154 L114 | L154 L114 L111 L152 | L114 L69 L113 L156 | L244 L226 L243 L21 | L22 L193 L192 L249 | L254 L192 L248 L71 | L255 L195 L254 L192 | L192 L197 L195 L255 | L235 L71 L70 L238 | L154 L113 L111 L114 | L156 L153 L78 L113 | L113 L69 L68 L150 L156 | L243 L226 L230 L193 | L192 L196 L195 L197 | L248 L192 L231 L71 | L254 L195 L248 L192 | L173 A46 L17 L113 L154 | L78 L153 L10 A74 L49 | L150 L68 L78 L153 | L230 L226 L227 L196 | L248 L195 L231 L192 | L154 L153 L17 L112 L111 L113 | L113 L165 A45 L166 L17 L153 L154 | L173 A47 A46 | A46 L173 A47 | L50 L12 L153 L77 A70 | L77 A70 L153 L17 L113 | L10 A74 L153 L169 A56 L14 | L78 L67 L10 L153 | L113 L17 L166 A45 L165 | L173 A47 | A47 L173 | L14 L169 A56 L153 L12 | A70 L77 | L77 A70 | A74 L10 | L10 A74 | L10 L11 L12 L153 | L165 A60 L166 A45 | A45 L166 A60 L165 | L153 L77 L18 L17 | L12 L18 L77 L153 | A60 L166 A44 L165 | L165 A44 L166 A60 | A56 L169 A57 | L169 A57 A56 | L165 L166 A44 | A44 L166 L165 | A57 L169 | L169 A57 | A48 | A49 | A50 | A51 | A52 | A53 | A54 | A55 | A58 | A59 | A61 | A62 | A63 | A64 | A65 | A66 | A67 | A68 | A69 | A71 | A72 | A73 | A75 | A76 | A77 | A78 | A79 | A80 | A81 | A82 | A83 | A84 | A85 | A86 | A87
extrude "wire pass through" cut sketch "Sketch2" along normal blind 2 contours L3 L2 L229 L0 | L4 L155 L12 L3 | L229 L2 L242 L0 | L12 L155 L17 L3 | L4 A88 L15 L12 L155 | L12 L114 L17 L155 | L4 A88 | L1 L240 L22 L19 | L22 L249 L192 L255 | L192 L197 L195 L255 | A58 | A59 | A83 | A84 | A85 | A86 | A87 picked at (-5.8995, 1.9409)
extrude "enclosure hinges" add sketch "Sketch2" against normal blind 4.8 from surface at 8.2 contours L114 L104 L215 L69 | L69 L206 L104 L113 | L233 L104 L219 L69 | L69 L210 L104 L232
chamfer "Chamfer1" distance 2 angle 45 2 edges at (55.2, -7.6, 0) (55.2, 69.4, 0)
body "Solid1"
